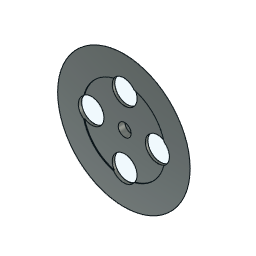
Bächerhalter v2 (Autodesk Fusion 360 design; units mm, degrees)
Autodesk Fusion 360 part; units mm, degrees
sketch "Skizze1" plane through (0, 0, 0) normal (0, 1, 0) x (1, 0, 0)
  circle A0 centre (0, 0) radius 40
  dimension "d1" = 80
  constraint coincident A0.centre origin
  measures "d1" diameter of A0
extrude "Extrusion1" add sketch "Skizze1" along normal blind 2
sketch "Skizze2" plane through (0, 2, 0) normal (0, 1, 0) x (-1, 0, 0)
  circle A0 centre (0, 0) radius 40
  circle A1 centre (0, 0) radius 4
  dimension "d4" = 8
  constraint coincident A0.centre A1.centre
  measures "d4" diameter of A1
extrude "Extrusion2" add sketch "Skizze2" along normal blind 1 contours A1
extrude "Extrusion3" add 1 faces at (1.2456, 3, 0.0132) along direction (0, 1, 0) blind 2
fillet "Abrundung1" radius 40 1 edges at (-37.2931, 2, 14.4646)
hole "Bohrung1" at (0, 0, 0) direction (0, 1, 0) diameter 0.9 depth 100 tip angle 180 counterbore diameter 7.8 counterbore depth 4.5
move_face "Flächen versetzen1" offset 0.5 1 faces at (-3.995, 4, -0.1994)
sketch "Skizze3" plane through (0, 0, 0) normal (0, -1, 0) x (1, 0, 0)
  circle A0 centre (0, 0) radius 3.9
  circle A1 centre (0, 0) radius 40
  circle A2 centre (-20, 0) radius 7.5
  circle A3 centre (0, 20) radius 7.5
  circle A4 centre (19.9998, -0.0933) radius 7.5
  circle A5 centre (-0.0227, -20) radius 7.5
  dimension "d17" = 15
  dimension "d18" = 15
  dimension "d19" = 15
  dimension "d20" = 15
  dimension "d21" = 20
  dimension "d22" = 20
  dimension "d23" = 20
  dimension "d24" = 20
  measures "d17" diameter of A2
  measures "d18" diameter of A3
  measures "d19" diameter of A4
  measures "d20" diameter of A5
  measures "d21" distance of A0.centre A5.centre
  measures "d22" distance of A0.centre A4.centre
  measures "d23" distance of A0.centre A3.centre
  measures "d24" distance of A0.centre A2.centre
extrude "Extrusion4" cut sketch "Skizze3" against normal blind 21 contours A2 | A3 | A4 | A5
sketch "Skizze4" plane through (0, 0, 0) normal (0, -1, 0) x (1, 0, 0)
  circle A0 centre (0, 20) radius 7.5
  circle A1 centre (19.9998, -0.0933) radius 7.5
  circle A2 centre (-20, 0) radius 7.5
  circle A3 centre (-0.0227, -20) radius 7.5
  circle A4 centre (0, 0) radius 3.9
  circle A5 centre (0, 0) radius 40
  circle A6 centre (0, 0) radius 25
  dimension "d27" = 50
  constraint concentric A4 A6
  measures "d27" diameter of A6
extrude "Extrusion5" cut sketch "Skizze4" against normal blind 0.5 contours A0 A1 A2 A3 A6
sketch "Skizze5" plane through (0, 0, 0) normal (0, -1, 0) x (1, 0, 0)
  arc A0 (6.1735, -24.2258) -> (24.1895, -6.3139) centre (0, 0) ccw
  arc A1 (-6.2285, -24.2117) -> (6.1735, -24.2258) centre (-0.0227, -20) ccw
  arc A2 (-24.2188, -6.201) -> (-6.2285, -24.2117) centre (0, 0) ccw
  arc A3 (-24.2188, 6.201) -> (-24.2188, -6.201) centre (-20, 0) ccw
  arc A4 (-6.201, 24.2188) -> (-24.2188, 6.201) centre (0, 0) ccw
  arc A5 (6.201, 24.2188) -> (-6.201, 24.2188) centre (0, 20) ccw
  arc A6 (24.2474, 6.0879) -> (6.201, 24.2188) centre (0, 0) ccw
  arc A7 (24.1895, -6.3139) -> (24.2474, 6.0879) centre (19.9998, -0.0933) ccw
  circle A8 centre (0, 0) radius 40
